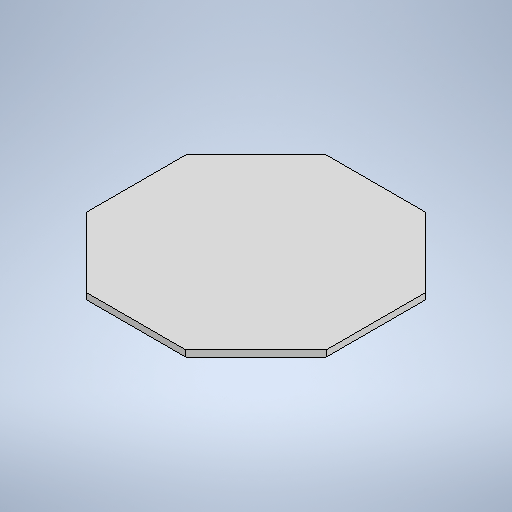
# Autodesk Inventor part: 210 DS-B Axis cap
Saved by Autodesk Inventor 2025 (Build 290162010, 162A)
## iProperties
Created: 2024-12-09
Part Number: 210 DS-B Axis cap
Material: Stainless Steel
Document SubType Name: Sheet Metal
Designer: admin
Mass: 344.52 g
Surface Area: 230.435 cm^2
Volume: 43.065 cm^3
Density: 8 g/cm^3
Flat Pattern Width: 11.4 cm
Flat Pattern Length: 11.4 cm
Flat Pattern Area: 129.96 cm^2
Sheet Metal Rule: AISI304 3mm Die 32
Sheet Metal Width: 114,000 mm
Sheet Metal Length: 114,000 mm
Sheet Metal Area: 12996,000 mm^2
Appearance: Default
Author: user
Autodesk Inventor part; units mm, degrees
ref_plane "YZ Plane" through (0, 0, 0) normal (1, 0, 0) x (0, 1, 0)
ref_plane "XZ Plane" through (0, 0, 0) normal (0, 1, 0) x (-1, 0, 0)
ref_plane "XY Plane" through (0, 0, 0) normal (0, 0, 1) x (1, 0, 0)
sketch "Sketch1" plane through (0, 0, 0) normal (0, 0, 1) x (1, 0, 0)
  circle A0 centre (0, 0) radius 57 construction
  circle A1 centre (0, 0) radius 105 construction
  line L0 (105, -105) -> (-105, -105)
  line L1 (-105, -105) -> (-105, 105)
  line L2 (-105, 105) -> (105, 105)
  line L3 (105, 105) -> (105, -105)
  line L4 (105, -105) -> (-105, 105) construction
  line L5 (-105, -105) -> (105, 105) construction
  line L6 (43.4924, 105) -> (105, 43.4924)
  line L7 (105, 43.4924) -> (105, -43.4924)
  line L8 (105, -43.4924) -> (43.4924, -105)
  line L9 (43.4924, -105) -> (-43.4924, -105)
  line L10 (-43.4924, -105) -> (-105, -43.4924)
  line L11 (-105, -43.4924) -> (-105, 43.4924)
  line L12 (-105, 43.4924) -> (-43.4924, 105)
  line L13 (-43.4924, 105) -> (43.4924, 105)
  line L14 (23.6102, 57) -> (57, 23.6102)
  line L15 (57, 23.6102) -> (57, -23.6102)
  line L16 (57, -23.6102) -> (23.6102, -57)
  line L17 (23.6102, -57) -> (-23.6102, -57)
  line L18 (-23.6102, -57) -> (-57, -23.6102)
  line L19 (-57, -23.6102) -> (-57, 23.6102)
  line L20 (-57, 23.6102) -> (-23.6102, 57)
  line L21 (-23.6102, 57) -> (23.6102, 57)
  point P0 (0, 105)
  point P1 (-105, 43.4924)
  point P2 (-43.4924, -105)
  point P3 (0, 57)
  dimension "d22" = 114
  dimension "d23" = 210
extrude "Plate1" add sketch "Sketch1" along normal blind 3 contours L14 L15 L16 L17 L18 L19 L20 L21
sketch "Sketch6" plane through (0, 0, 0) normal (0, 0, 1) x (1, 0, 0)
  line L0 (0, 0) -> (0, 85) construction
  circle A0 centre (0, 0) radius 85 construction
  line L1 (0, 0) -> (60.1041, 60.1041) construction
  circle A1 centre (60.1041, 60.1041) radius 9
  dimension "d32" = 18
  dimension "d33" = 170
  dimension "d34" = 45
  constraints: 4 end point, 2 centre point, 2 coincident, 2 point on circle, 1 vertical
  measures "d32" diameter of A1
  measures "d33" diameter of A0
  measures "d34" angle of L0 L1
cut "Cut2" [suppressed]
pattern_circular "Circular Pattern2" [suppressed]
equation "\"d23\" = Flange_D_outer"
equation "\"d32\" = Flange_d_hole_diam"
equation "\"d33\" = Flange_D1_hole_center"
equation "\"d35\" = Thickness"
equation "\"d2\" = Thickness"
equation "\"BendReliefWidth\" = Thickness"
equation "\"BendReliefDepth\" = 0.5 * Thickness"
equation "\"CornerReliefSize\" = 4 * Thickness"
equation "\"MinimumRemnant\" = 2 * Thickness"
equation "\"TransitionRadius\" = BendRadius"
equation "\"JacobiRadiusSize\" = BendRadius"
equation "\"GapSize\" = Thickness"
equation "\"Flange_D_outer\" = 210"
equation "\"Flange_d_hole_diam\" = 18"
equation "\"Flange_D1_hole_center\" = 170"
equation "\"Thickness\" = 3"
equation "\"BendRadius\" = 5"
body "Solid1"
